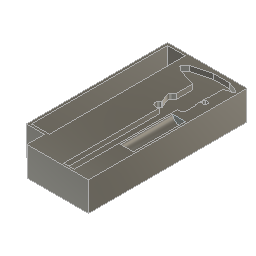
Dial-Caliper-Carrier (Autodesk Fusion 360 design; units mm, degrees)
Autodesk Fusion 360 part; units mm, degrees
(part 1 of 2)
sketch "Sketch1" plane through (0, 0, 3.175) normal (0, 0, 1) x (-1, 0, 0)
  line L0 (0, 0) -> (0, 297.942)
  line L1 (0, 297.942) -> (-407.924, 297.942)
  line L2 (-407.924, 297.942) -> (-407.924, 0)
  line L3 (-407.924, 0) -> (0, 0)
  line L4 (-407.924, 0) -> (-312.924, 0)
  line L5 (-312.924, 0) -> (-312.924, 245)
  line L6 (-312.924, 245) -> (-407.924, 245)
  line L7 (-407.924, 245) -> (-407.924, 0)
  dimension "d206" = 95
  dimension "d207" = 245
  constraint horizontal L4
  constraint vertical L5
  constraint horizontal L6
  constraint vertical L7
  constraint coincident L2.end L3.start
  measures "d206" distance of L2.end L4.end
  measures "d207" distance of L2.end L6.end
extrude "Extrude1" add sketch "Sketch1" along normal blind 45 contours L2 L3 L4 L5 L6 L7
sketch "Sketch2" plane through (0, 0, 48.175) normal (0, 0, 1) x (-1, 0, 0)
  line L0 (-407.924, 245) -> (-407.924, 0)
  line L1 (-407.924, 0) -> (-312.924, 0)
  line L2 (-312.924, 0) -> (-312.924, 245)
  line L3 (-312.924, 245) -> (-407.924, 245)
sketch "Sketch3" plane through (0, 0, 48.175) normal (0, 0, 1) x (-1, 0, 0)
  line L0 (-385.7159, 241.3097) -> (-385.7159, 82.3904)
  line L1 (-312.924, 245) -> (-407.924, 245)
  line L2 (-407.924, 245) -> (-407.924, 0)
  line L3 (-317.924, 240) -> (-317.924, 87.6)
  line L4 (-312.924, 0) -> (-312.924, 245)
  line L5 (-317.924, 87.6) -> (-336.974, 87.6)
  line L6 (-336.974, 87.6) -> (-336.974, 240)
  line L7 (-336.974, 240) -> (-317.924, 240)
  line L8 (-337.024, 240.05) -> (-317.874, 240.05)
  line L9 (-317.874, 240.05) -> (-317.874, 87.55)
  line L10 (-317.874, 87.55) -> (-337.024, 87.55)
  line L11 (-337.024, 87.55) -> (-337.024, 240.05)
  dimension "d210" = 152.4
  dimension "d211" = 5
  dimension "d212" = 5
  dimension "d213" = 19.05
  dimension "d214" = -0.05
  constraint parallel L0 L2
  constraint perpendicular L1 L3
  constraint perpendicular L3 L5
  constraint perpendicular L5 L6
  constraint perpendicular L3 L7
  measures "d210" distance of L3.start L3.end
  measures "d211" distance of L3 L4
  measures "d212" distance of L1 L3.start
  measures "d213" distance of L3.end L5.end
sketch "Sketch5" plane through (0, 0, 48.175) normal (0, 0, 1) x (-1, 0, 0)
  line L0 (-407.924, 245) -> (-407.924, 0)
  line L1 (-407.924, 0) -> (-312.924, 0)
  line L2 (-312.924, 0) -> (-312.924, 245)
  line L3 (-312.924, 245) -> (-407.924, 245)
  line L4 (-366.4147, 241.7185) -> (-366.3062, 93.0229)
  line L5 (-366.4147, 241.7185) -> (-382.673, 241.7066)
  line L6 (-382.673, 241.7066) -> (-382.5568, 82.4778)
  spline S0 degree 5 poles (-382.5568, 82.4778) (-382.5593, 82.4568) (-382.563, 82.4147) (-382.5646, 82.3519) (-382.559, 82.2687) (-382.5488, 82.169) (-382.5684, 82.0854) (-382.6594, 82.0319) (-382.8401, 82.0111) (-383.1037, 82.0144) (-383.4312, 82.0288) (-383.8005, 82.0428) (-384.1971, 82.0514) (-384.6109, 82.0543) (-385.0359, 82.0538) (-385.4676, 82.0533) (-385.9022, 82.0552) (-386.3345, 82.0591) (-386.7578, 82.0608) (-387.165, 82.0543) (-387.5495, 82.0319) (-387.9064, 81.9855) (-388.2336, 81.9077) (-388.5328, 81.7926) (-388.8079, 81.6362) (-389.0641, 81.4368) (-389.306, 81.1959) (-389.5364, 80.9182) (-389.7556, 80.6117) (-389.9622, 80.2849) (-390.1543, 79.9453) (-390.3301, 79.5967) (-390.4889, 79.2371) (-390.6319, 78.8575) (-390.7613, 78.4459) (-390.8799, 77.9908) (-390.9902, 77.4855) (-391.0939, 76.9317) (-391.1914, 76.3431) (-391.2811, 75.7505) (-391.3598, 75.1937) (-391.4238, 74.7122) (-391.4698, 74.337) (-391.4957, 74.0802) (-391.5015, 73.9279) (-391.4903, 73.827) (-391.4674, 73.701) (-391.4381, 73.482) (-391.4063, 73.1351) (-391.3744, 72.6507) (-391.344, 72.0401) (-391.3158, 71.3289) (-391.2898, 70.5518) (-391.2656, 69.7464) (-391.243, 68.9483) (-391.2214, 68.1843) (-391.2007, 67.4704) (-391.1809, 66.8139) (-391.1621, 66.2157) (-391.1444, 65.6712) (-391.1281, 65.1725) (-391.1133, 64.7103) (-391.1002, 64.2749) (-391.0891, 63.8589) (-391.0801, 63.4574) (-391.0732, 63.0673) (-391.0693, 62.7632) (-391.0674, 62.5394) (-391.0665, 62.3921) (-391.0662, 62.3189) knots 0 0 0 0 0 0 0.01538462 0.03076923 0.04615385 0.06153846 0.07692308 0.09230769 0.10769231 0.12307692 0.13846154 0.15384615 0.16923077 0.18461538 0.2 0.21538462 0.23076923 0.24615385 0.26153846 0.27692308 0.29230769 0.30769231 0.32307692 0.33846154 0.35384615 0.36923077 0.38461538 0.4 0.41538462 0.43076923 0.44615385 0.46153846 0.47692308 0.49230769 0.50769231 0.52307692 0.53846154 0.55384615 0.56923077 0.58461538 0.6 0.61538462 0.63076923 0.64615385 0.66153846 0.67692308 0.69230769 0.70769231 0.72307692 0.73846154 0.75384615 0.76923077 0.78461538 0.8 0.81538462 0.83076923 0.84615385 0.86153846 0.87692308 0.89230769 0.90769231 0.92307692 0.93846154 0.95384615 0.96923077 0.98461538 1 1 1 1 1 1
  spline S1 degree 5 poles (-389.9505, 61.1725) (-389.9505, 61.0932) (-389.9505, 60.9369) (-389.9505, 60.7095) (-389.9505, 60.42) (-389.9505, 60.0804) (-389.9505, 59.7592) (-389.9505, 59.4492) (-389.9505, 59.1366) (-389.9505, 58.8031) (-389.9505, 58.4302) (-389.9505, 58.0029) (-389.9505, 57.5144) (-389.9505, 56.97) (-389.9505, 56.385) (-389.9505, 55.7806) (-389.9505, 55.1811) (-389.9505, 54.6105) (-389.9505, 54.0894) (-389.9505, 53.6317) (-389.9505, 53.2443) (-389.9505, 52.993) (-389.9505, 52.8376) (-389.9505, 52.7487) (-389.9505, 52.7079) knots 0 0 0 0 0 0 0.05 0.1 0.15 0.2 0.25 0.3 0.35 0.4 0.45 0.5 0.55 0.6 0.65 0.7 0.75 0.8 0.85 0.9 0.95 1 1 1 1 1 1
  spline S2 degree 5 poles (-391.075, 63.1525) (-391.0747, 63.1374) (-391.0729, 63.1049) (-391.0668, 63.0492) (-391.0519, 62.9611) (-391.0219, 62.828) (-390.9803, 62.6732) (-390.927, 62.4996) (-390.8622, 62.3125) (-390.7861, 62.1204) (-390.6996, 61.933) (-390.6038, 61.7602) (-390.5004, 61.6101) (-390.3919, 61.4876) (-390.2816, 61.3926) (-390.1737, 61.3196) (-390.0836, 61.2661) (-390.0205, 61.2265) (-389.9798, 61.1969) (-389.9574, 61.1784) (-389.9505, 61.1725) knots 0 0 0 0 0 0 0.05 0.1 0.15 0.2 0.25 0.3 0.35 0.4 0.45 0.5 0.55 0.6 0.65 0.7 0.75 0.77292 0.77292 0.77292 0.77292 0.77292 0.77292
  line L7 (-390.106, 61.306) -> (-389.795, 61.0389)
  spline S3 degree 5 poles (-387.4662, 6.0325) (-386.4601, 6.0325) (-384.4479, 6.0325) (-381.4296, 6.0325) (-377.4051, 6.0325) (-372.3746, 6.0325) (-368.3502, 6.0325) (-365.3319, 6.0325) (-363.3197, 6.0325) (-362.3136, 6.0325) knots 0 0 0 0 0 0 0.2 0.4 0.6 0.8 1 1 1 1 1 1
  spline S4 degree 5 poles (-362.3136, 6.0325) (-362.1526, 6.0601) (-361.8173, 6.1205) (-361.274, 6.2265) (-360.4685, 6.3988) (-359.3264, 6.6655) (-358.0528, 6.9821) (-356.6573, 7.3442) (-355.1586, 7.7439) (-353.5804, 8.1713) (-351.9486, 8.6156) (-350.2888, 9.0666) (-348.6228, 9.5161) (-346.9663, 9.9592) (-345.3286, 10.394) (-343.7147, 10.8206) (-342.1264, 11.2407) (-340.5633, 11.6563) (-339.0245, 12.0695) (-337.5089, 12.4816) (-336.0158, 12.8932) (-334.8388, 13.2226) (-333.9657, 13.4696) (-333.3878, 13.6343) (-333.1, 13.7167) knots 0 0 0 0 0 0 0.05 0.1 0.15 0.2 0.25 0.3 0.35 0.4 0.45 0.5 0.55 0.6 0.65 0.7 0.75 0.8 0.85 0.9 0.95 1 1 1 1 1 1
  spline S5 degree 5 poles (-333.1, 13.7167) (-332.8186, 14.0144) (-332.2556, 14.6098) (-331.4112, 15.503) (-330.2854, 16.6939) (-328.8781, 18.1825) (-327.7522, 19.3734) (-326.9078, 20.2666) (-326.3449, 20.862) (-326.0635, 21.1597) knots 0 0 0 0 0 0 0.2 0.4 0.6 0.8 1 1 1 1 1 1
  spline S6 degree 5 poles (-326.0635, 21.1597) (-326.0507, 21.1722) (-326.0252, 21.197) (-325.9869, 21.2343) (-325.9359, 21.284) (-325.8721, 21.3461) (-325.821, 21.3957) (-325.7827, 21.433) (-325.7572, 21.4578) (-325.7445, 21.4703) knots 0 0 0 0 0 0 0.2 0.4 0.6 0.8 1 1 1 1 1 1
  spline S7 degree 5 poles (-332.3207, 27.7023) (-332.0446, 27.4406) (-331.4923, 26.9172) (-330.6638, 26.1321) (-329.5592, 25.0853) (-328.2439, 23.8389) (-327.2048, 22.8542) (-326.4419, 22.1312) (-325.9551, 21.6699) (-325.7445, 21.4703) knots 0 0 0 0 0 0 0.2 0.4 0.6 0.8 0.95254 0.95254 0.95254 0.95254 0.95254 0.95254
  line L8 (-326.4152, 22.1059) -> (-325.0737, 20.8346)
  line L9 (-332.3207, 27.7023) -> (-359.9697, 35.6695)
  line L10 (-359.9697, 35.6695) -> (-359.9697, 43.0263)
  line L11 (-359.9697, 43.0263) -> (-359.9697, 61.0097)
  spline S8 degree 5 poles (-359.9697, 61.0097) (-359.9018, 61.0819) (-359.7646, 61.2258) (-359.5543, 61.4403) (-359.2647, 61.7233) (-358.8875, 62.0728) (-358.4957, 62.4196) (-358.0905, 62.7671) (-357.674, 63.1207) (-357.2495, 63.4874) (-356.8218, 63.8741) (-356.3978, 64.2876) (-355.9865, 64.7329) (-355.5989, 65.2134) (-355.2464, 65.7307) (-354.9403, 66.2847) (-354.6905, 66.8732) (-354.5054, 67.4925) (-354.391, 68.1384) (-354.3516, 68.808) (-354.3894, 69.5005) (-354.5046, 70.219) (-354.6951, 70.9706) (-354.9569, 71.7634) (-355.2837, 72.6045) (-355.6671, 73.4983) (-356.0968, 74.4439) (-356.5602, 75.4327) (-357.0428, 76.4482) (-357.5291, 77.4686) (-358.0035, 78.4687) (-358.4508, 79.4224) (-358.8574, 80.3045) (-359.2118, 81.0929) (-359.5055, 81.771) (-359.7337, 82.3297) (-359.8622, 82.6775) (-359.9278, 82.8821) (-359.958, 82.9935) (-359.9697, 83.043) knots 0 0 0 0 0 0 0.028571 0.057143 0.085714 0.114286 0.142857 0.171429 0.2 0.228571 0.257143 0.285714 0.314286 0.342857 0.371429 0.4 0.428571 0.457143 0.485714 0.514286 0.542857 0.571429 0.6 0.628571 0.657143 0.685714 0.714286 0.742857 0.771429 0.8 0.828571 0.857143 0.885714 0.914286 0.942857 0.971429 1 1 1 1 1 1
  spline S9 degree 5 poles (-359.9697, 83.043) (-359.8778, 83.0783) (-359.6942, 83.1489) (-359.4187, 83.2549) (-359.0514, 83.3961) (-358.5923, 83.5727) (-358.2249, 83.7139) (-357.9495, 83.8198) (-357.7658, 83.8905) (-357.674, 83.9258) knots 0 0 0 0 0 0 0.2 0.4 0.6 0.8 1 1 1 1 1 1
  spline S10 degree 5 poles (-359.9697, 83.043) (-359.9166, 83.0639) (-359.81, 83.1056) (-359.6489, 83.1679) (-359.4317, 83.2503) (-359.1558, 83.3538) (-358.8752, 83.4625) (-358.5893, 83.5858) (-358.2969, 83.7381) (-357.9979, 83.9346) (-357.6939, 84.1868) (-357.389, 84.4988) (-357.091, 84.8639) (-356.8092, 85.2687) (-356.553, 85.6961) (-356.3303, 86.1297) (-356.1458, 86.5564) (-355.9991, 86.9709) (-355.8859, 87.3747) (-355.8004, 87.7738) (-355.7373, 88.1762) (-355.6936, 88.5902) (-355.6713, 89.0222) (-355.6759, 89.4755) (-355.7154, 89.9513) (-355.798, 90.4477) (-355.9313, 90.9599) (-356.1199, 91.4799) (-356.3653, 91.9969) (-356.6667, 92.4989) (-357.0208, 92.9738) (-357.4229, 93.4106) (-357.8674, 93.8004) (-358.3475, 94.1384) (-358.8567, 94.4239) (-359.3882, 94.6593) (-359.9353, 94.848) (-360.4919, 94.9934) (-361.0522, 95.0971) (-361.6114, 95.1576) (-362.1658, 95.1683) (-362.712, 95.1199) (-363.2471, 95.0039) (-363.7673, 94.8157) (-364.2682, 94.5576) (-364.7435, 94.2418) (-365.1849, 93.8948) (-365.5824, 93.5536) (-365.8932, 93.2873) (-366.0959, 93.134) (-366.2188, 93.0608) (-366.2846, 93.0312) (-366.3062, 93.0229) knots 0 0 0 0 0 0 0.02 0.04 0.06 0.08 0.1 0.12 0.14 0.16 0.18 0.2 0.22 0.24 0.26 0.28 0.3 0.32 0.34 0.36 0.38 0.4 0.42 0.44 0.46 0.48 0.5 0.52 0.54 0.56 0.58 0.6 0.62 0.64 0.66 0.68 0.7 0.72 0.74 0.76 0.78 0.8 0.82 0.84 0.86 0.88 0.9 0.92 0.94 0.950494 0.950494 0.950494 0.950494 0.950494 0.950494
  line L12 (-365.399, 93.3737) -> (-367.2134, 92.6721)
  line L13 (-387.8522, 7.1354) -> (-387.8522, 6.0325)
  line L14 (-387.8522, 6.0325) -> (-387.4662, 6.0325)
  line L15 (-387.8522, 6.8243) -> (-400.7794, 11.0064)
  line L16 (-400.7794, 11.0064) -> (-404.4624, 13.6097)
  line L17 (-404.4624, 13.6097) -> (-401.1196, 16.5087)
  line L18 (-401.1196, 16.5087) -> (-390.396, 19.9107)
  arc A0 (-390.396, 19.9107) -> (-390.6158, 20.6037) centre (-390.5059, 20.2572) ccw
  line L19 (-390.6158, 20.6037) -> (-390.6158, 41.3132)
  line L20 (-390.6158, 48.1829) -> (-396.3987, 48.1829)
  spline S11 degree 5 poles (-391.5467, 48.1829) (-391.5195, 48.185) (-391.4654, 48.1911) (-391.3847, 48.2058) (-391.2783, 48.2369) (-391.1473, 48.2953) (-391.0189, 48.374) (-390.8943, 48.4742) (-390.7753, 48.5968) (-390.6642, 48.7426) (-390.5636, 48.9124) (-390.4762, 49.1069) (-390.4037, 49.326) (-390.3474, 49.5695) (-390.3073, 49.8363) (-390.2832, 50.1256) (-390.2765, 50.3743) (-390.2784, 50.5702) (-390.2828, 50.705) (-390.2857, 50.7734) knots 0 0 0 0 0 0 0.066667 0.133333 0.2 0.266667 0.333333 0.4 0.466667 0.533333 0.6 0.666667 0.733333 0.8 0.866667 0.933333 1 1 1 1 1 1
  spline S12 degree 5 poles (-390.2857, 52.3633) (-390.2961, 52.4211) (-390.3173, 52.5354) (-390.3502, 52.7038) (-390.3967, 52.9217) (-390.4591, 53.1824) (-390.5263, 53.4305) (-390.5987, 53.6646) (-390.6766, 53.8841) (-390.7599, 54.0891) (-390.8482, 54.2808) (-390.9226, 54.4242) (-390.9803, 54.5265) (-391.0196, 54.5925) (-391.0395, 54.6249) knots 0 0 0 0 0 0 0.1 0.2 0.3 0.4 0.5 0.6 0.7 0.8 0.9 1 1 1 1 1 1
  spline S13 degree 5 poles (-391.0395, 54.6249) (-391.1432, 54.6249) (-391.3521, 54.6249) (-391.6698, 54.6249) (-392.102, 54.6249) (-392.6578, 54.6249) (-393.2304, 54.6249) (-393.8211, 54.6249) (-394.4301, 54.6249) (-395.0566, 54.6249) (-395.6991, 54.6249) (-396.2247, 54.6249) (-396.6251, 54.6249) (-396.8947, 54.6249) (-397.0302, 54.6249) knots 0 0 0 0 0 0 0.1 0.2 0.3 0.4 0.5 0.6 0.7 0.8 0.9 1 1 1 1 1 1
  spline S14 degree 5 poles (-397.0302, 54.6249) (-397.06, 54.605) (-397.1182, 54.5641) (-397.2016, 54.4991) (-397.3046, 54.4051) (-397.4199, 54.2753) (-397.5222, 54.1324) (-397.6123, 53.9753) (-397.6921, 53.8022) (-397.7634, 53.611) (-397.8286, 53.3999) (-397.8892, 53.168) (-397.946, 52.916) (-397.9988, 52.6463) (-398.0463, 52.3623) (-398.0869, 52.0681) (-398.1183, 51.7675) (-398.1381, 51.4639) (-398.1438, 51.1591) (-398.1331, 50.8546) (-398.104, 50.551) (-398.0548, 50.2496) (-397.9848, 49.952) (-397.8939, 49.6613) (-397.7831, 49.3821) (-397.6541, 49.1201) (-397.5092, 48.8811) (-397.3504, 48.6711) (-397.1797, 48.4948) (-396.9988, 48.3556) (-396.8084, 48.2552) (-396.6489, 48.2065) (-396.5253, 48.1877) (-396.4412, 48.1832) (-396.3987, 48.1829) knots 0 0 0 0 0 0 0.033333 0.066667 0.1 0.133333 0.166667 0.2 0.233333 0.266667 0.3 0.333333 0.366667 0.4 0.433333 0.466667 0.5 0.533333 0.566667 0.6 0.633333 0.666667 0.7 0.733333 0.766667 0.8 0.833333 0.866667 0.9 0.933333 0.966667 1 1 1 1 1 1
  line L21 (-390.2857, 50.7734) -> (-389.869, 50.7734)
  line L22 (-389.869, 50.7734) -> (-389.869, 42.5841)
  line L23 (-389.869, 42.5841) -> (-390.6158, 41.3132)
  line L24 (-390.2857, 52.3633) -> (-389.9496, 52.3633)
  line L25 (-389.9496, 52.3633) -> (-389.9505, 52.7079)
  point P0 (-382.5566, 82.2421)
  point P1 (-382.6149, 82.068)
  point P2 (-383.4158, 82.0278)
  point P3 (-385.6935, 82.0546)
  point P4 (-387.9176, 81.9742)
  point P5 (-389.2173, 81.2775)
  point P6 (-390.3025, 79.6429)
  point P7 (-391.1064, 76.8426)
  point P8 (-391.495, 74.0424)
  point P9 (-391.4682, 73.6941)
  point P10 (-391.2538, 69.3262)
  point P11 (-391.1064, 64.4761)
  point P12 (-390.9289, 62.5109)
  point P13 (-390.428, 61.5325)
  point P14 (-389.9505, 59.6047)
  point P15 (-389.9505, 57.9413)
  point P16 (-389.9505, 54.4545)
  point P17 (-358.1946, 6.9498)
  point P18 (-349.922, 9.165)
  point P19 (-340.888, 11.5706)
  point P20 (-358.509, 62.4052)
  point P21 (-356.7435, 63.956)
  point P22 (-355.0257, 66.151)
  point P23 (-354.3815, 69.1811)
  point P24 (-355.9084, 74.0244)
  point P25 (-359.1532, 80.9673)
  point P26 (-358.9561, 83.4328)
  point P27 (-357.7318, 84.1668)
  point P28 (-356.2907, 86.2339)
  point P29 (-355.7325, 88.2562)
  point P30 (-355.8698, 90.6995)
  point P31 (-357.7915, 93.7193)
  point P32 (-361.159, 95.1011)
  point P33 (-364.3984, 94.4606)
  point P34 (-390.971, 48.4159)
  point P35 (-390.4638, 49.156)
  point P36 (-390.6154, 53.7066)
  point P37 (-393.7051, 54.6249)
  point P38 (-397.5325, 54.1077)
  point P39 (-397.8674, 53.2466)
  point P40 (-398.1186, 51.7276)
  point P41 (-397.987, 49.9813)
  point P42 (-397.2813, 48.6058)
  constraint perpendicular L4 L5
  constraint perpendicular L5 L6
  constraint coincident S0 S2.start
  constraint coincident S1.start S2.end
  constraint midpoint S1.start L7
  constraint midpoint S6.end L8
  constraint vertical L10
  constraint parallel L10 L11
  constraint coincident S9 P26
  constraint midpoint L4.end L12
  constraint vertical L13
  constraint perpendicular L13 L14
  constraint coincident L13 L15.start
  constraint tangent L18 A0
  constraint vertical L19
  constraint perpendicular L19 L20
  constraint coincident L20 S11.start
  constraint horizontal L21
  constraint perpendicular L21 L22
  constraint perpendicular L19 L24
extrude "Extrude4" cut sketch "Sketch5" against normal blind 8 contours L4 L5 L6 S0 S1 S2 S3 S4 S5 S6 S7 L8 L9 L10 L11 S8 S10 L13 L14 L15 L16 L17 L18 A0 L19 L20 S11 S12 S13 S14 L21 L22 L23 L24 L25
sketch "Sketch11" plane through (0, 0, 48.175) normal (0, 0, 1) x (-1, 0, 0)
  line L0 (-362.3136, 6.0325) -> (-387.8522, 6.0325)
  line L1 (-387.8522, 6.0325) -> (-387.8522, 6.8243)
  line L2 (-387.8522, 6.8243) -> (-400.7794, 11.0064)
  line L3 (-400.7794, 11.0064) -> (-404.4624, 13.6097)
  line L4 (-404.4624, 13.6097) -> (-401.1196, 16.5087)
  line L5 (-401.1196, 16.5087) -> (-390.396, 19.9107)
  arc A0 (-390.396, 19.9107) -> (-390.6158, 20.6037) centre (-390.5059, 20.2572) ccw
  line L6 (-390.6158, 20.6037) -> (-390.6158, 41.3132)
  line L7 (-390.6158, 41.3132) -> (-389.869, 42.5841)
  line L8 (-389.869, 42.5841) -> (-389.869, 50.7734)
  line L9 (-389.869, 50.7734) -> (-390.2857, 50.7734)
  spline S0 degree 5 poles (-390.2857, 50.7734) (-390.2828, 50.705) (-390.2784, 50.5702) (-390.2765, 50.3743) (-390.2832, 50.1256) (-390.3073, 49.8363) (-390.3474, 49.5695) (-390.4037, 49.326) (-390.4762, 49.1069) (-390.5636, 48.9124) (-390.6642, 48.7426) (-390.7753, 48.5968) (-390.8943, 48.4742) (-391.0189, 48.374) (-391.1473, 48.2953) (-391.2783, 48.2369) (-391.3847, 48.2058) (-391.4654, 48.1911) (-391.5195, 48.185) (-391.5467, 48.1829) knots -1 -1 -1 -1 -1 -1 -0.933333 -0.866667 -0.8 -0.733333 -0.666667 -0.6 -0.533333 -0.466667 -0.4 -0.333333 -0.266667 -0.2 -0.133333 -0.066667 0 0 0 0 0 0
  line L10 (-391.5467, 48.1829) -> (-396.3987, 48.1829)
  spline S1 degree 5 poles (-396.3987, 48.1829) (-396.4412, 48.1832) (-396.5253, 48.1877) (-396.6489, 48.2065) (-396.8084, 48.2552) (-396.9988, 48.3556) (-397.1797, 48.4948) (-397.3504, 48.6711) (-397.5092, 48.8811) (-397.6541, 49.1201) (-397.7831, 49.3821) (-397.8939, 49.6613) (-397.9848, 49.952) (-398.0548, 50.2496) (-398.104, 50.551) (-398.1331, 50.8546) (-398.1438, 51.1591) (-398.1381, 51.4639) (-398.1183, 51.7675) (-398.0869, 52.0681) (-398.0463, 52.3623) (-397.9988, 52.6463) (-397.946, 52.916) (-397.8892, 53.168) (-397.8286, 53.3999) (-397.7634, 53.611) (-397.6921, 53.8022) (-397.6123, 53.9753) (-397.5222, 54.1324) (-397.4199, 54.2753) (-397.3046, 54.4051) (-397.2016, 54.4991) (-397.1182, 54.5641) (-397.06, 54.605) (-397.0302, 54.6249) knots -1 -1 -1 -1 -1 -1 -0.966667 -0.933333 -0.9 -0.866667 -0.833333 -0.8 -0.766667 -0.733333 -0.7 -0.666667 -0.633333 -0.6 -0.566667 -0.533333 -0.5 -0.466667 -0.433333 -0.4 -0.366667 -0.333333 -0.3 -0.266667 -0.233333 -0.2 -0.166667 -0.133333 -0.1 -0.066667 -0.033333 0 0 0 0 0 0
  line L11 (-397.0302, 54.6249) -> (-391.0395, 54.6249)
  spline S2 degree 5 poles (-391.0395, 54.6249) (-391.0196, 54.5925) (-390.9803, 54.5265) (-390.9226, 54.4242) (-390.8482, 54.2808) (-390.7599, 54.0891) (-390.6766, 53.8841) (-390.5987, 53.6646) (-390.5263, 53.4305) (-390.4591, 53.1824) (-390.3967, 52.9217) (-390.3502, 52.7038) (-390.3173, 52.5354) (-390.2961, 52.4211) (-390.2857, 52.3633) knots -1 -1 -1 -1 -1 -1 -0.9 -0.8 -0.7 -0.6 -0.5 -0.4 -0.3 -0.2 -0.1 0 0 0 0 0 0
  line L12 (-390.2857, 52.3633) -> (-389.9496, 52.3633)
  line L13 (-389.9496, 52.3633) -> (-389.9505, 52.7079)
  line L14 (-389.9505, 52.7079) -> (-389.9505, 61.1725)
  spline S3 degree 5 poles (-389.9505, 61.1725) (-389.9574, 61.1784) (-389.9798, 61.1969) (-390.0205, 61.2265) (-390.0836, 61.2661) (-390.1737, 61.3196) (-390.2816, 61.3926) (-390.3919, 61.4876) (-390.5004, 61.6101) (-390.6038, 61.7602) (-390.6996, 61.933) (-390.7861, 62.1204) (-390.8622, 62.3125) (-390.927, 62.4996) (-390.9803, 62.6732) (-391.0219, 62.828) (-391.0519, 62.9611) (-391.0668, 63.0492) (-391.0729, 63.1049) (-391.0747, 63.1374) (-391.075, 63.1525) knots -0.77292 -0.77292 -0.77292 -0.77292 -0.77292 -0.77292 -0.75 -0.7 -0.65 -0.6 -0.55 -0.5 -0.45 -0.4 -0.35 -0.3 -0.25 -0.2 -0.15 -0.1 -0.05 0 0 0 0 0 0
  spline S4 degree 5 poles (-391.075, 63.1525) (-391.076, 63.2134) (-391.0784, 63.3525) (-391.0827, 63.5721) (-391.0896, 63.8767) (-391.1002, 64.2749) (-391.1133, 64.7103) (-391.1281, 65.1725) (-391.1444, 65.6712) (-391.1621, 66.2157) (-391.1809, 66.8139) (-391.2007, 67.4704) (-391.2214, 68.1843) (-391.243, 68.9483) (-391.2656, 69.7464) (-391.2898, 70.5518) (-391.3158, 71.3289) (-391.344, 72.0401) (-391.3744, 72.6507) (-391.4063, 73.1351) (-391.4381, 73.482) (-391.4674, 73.701) (-391.4903, 73.827) (-391.5015, 73.9279) (-391.4957, 74.0802) (-391.4698, 74.337) (-391.4238, 74.7122) (-391.3598, 75.1937) (-391.2811, 75.7505) (-391.1914, 76.3431) (-391.0939, 76.9317) (-390.9902, 77.4855) (-390.8799, 77.9908) (-390.7613, 78.4459) (-390.6319, 78.8575) (-390.4889, 79.2371) (-390.3301, 79.5967) (-390.1543, 79.9453) (-389.9622, 80.2849) (-389.7556, 80.6117) (-389.5364, 80.9182) (-389.306, 81.1959) (-389.0641, 81.4368) (-388.8079, 81.6362) (-388.5328, 81.7926) (-388.2336, 81.9077) (-387.9064, 81.9855) (-387.5495, 82.0319) (-387.165, 82.0543) (-386.7578, 82.0608) (-386.3345, 82.0591) (-385.9022, 82.0552) (-385.4676, 82.0533) (-385.0359, 82.0538) (-384.6109, 82.0543) (-384.1971, 82.0514) (-383.8005, 82.0428) (-383.4312, 82.0288) (-383.1037, 82.0144) (-382.8401, 82.0111) (-382.6594, 82.0319) (-382.5684, 82.0854) (-382.5488, 82.169) (-382.559, 82.2687) (-382.5646, 82.3519) (-382.563, 82.4147) (-382.5593, 82.4568) (-382.5568, 82.4778) knots -0.96593682 -0.96593682 -0.96593682 -0.96593682 -0.96593682 -0.96593682 -0.95384615 -0.93846154 -0.92307692 -0.90769231 -0.89230769 -0.87692308 -0.86153846 -0.84615385 -0.83076923 -0.81538462 -0.8 -0.78461538 -0.76923077 -0.75384615 -0.73846154 -0.72307692 -0.70769231 -0.69230769 -0.67692308 -0.66153846 -0.64615385 -0.63076923 -0.61538462 -0.6 -0.58461538 -0.56923077 -0.55384615 -0.53846154 -0.52307692 -0.50769231 -0.49230769 -0.47692308 -0.46153846 -0.44615385 -0.43076923 -0.41538462 -0.4 -0.38461538 -0.36923077 -0.35384615 -0.33846154 -0.32307692 -0.30769231 -0.29230769 -0.27692308 -0.26153846 -0.24615385 -0.23076923 -0.21538462 -0.2 -0.18461538 -0.16923077 -0.15384615 -0.13846154 -0.12307692 -0.10769231 -0.09230769 -0.07692308 -0.06153846 -0.04615385 -0.03076923 -0.01538462 0 0 0 0 0 0
  line L15 (-382.5568, 82.4778) -> (-382.673, 241.7066)
  line L16 (-382.673, 241.7066) -> (-366.4147, 241.7185)
  line L17 (-366.4147, 241.7185) -> (-366.3062, 93.0229)
  spline S5 degree 5 poles (-366.3062, 93.0229) (-366.2846, 93.0312) (-366.2188, 93.0608) (-366.0959, 93.134) (-365.8932, 93.2873) (-365.5824, 93.5536) (-365.1849, 93.8948) (-364.7435, 94.2418) (-364.2682, 94.5576) (-363.7673, 94.8157) (-363.2471, 95.0039) (-362.712, 95.1199) (-362.1658, 95.1683) (-361.6114, 95.1576) (-361.0522, 95.0971) (-360.4919, 94.9934) (-359.9353, 94.848) (-359.3882, 94.6593) (-358.8567, 94.4239) (-358.3475, 94.1384) (-357.8674, 93.8004) (-357.4229, 93.4106) (-357.0208, 92.9738) (-356.6667, 92.4989) (-356.3653, 91.9969) (-356.1199, 91.4799) (-355.9313, 90.9599) (-355.798, 90.4477) (-355.7154, 89.9513) (-355.6759, 89.4755) (-355.6713, 89.0222) (-355.6936, 88.5902) (-355.7373, 88.1762) (-355.8004, 87.7738) (-355.8859, 87.3747) (-355.9991, 86.9709) (-356.1458, 86.5564) (-356.3303, 86.1297) (-356.553, 85.6961) (-356.8092, 85.2687) (-357.091, 84.8639) (-357.389, 84.4988) (-357.6939, 84.1868) (-357.9979, 83.9346) (-358.2969, 83.7381) (-358.5478, 83.6074) (-358.7368, 83.5228) (-358.8668, 83.4687) (-358.9397, 83.4393) (-358.9561, 83.4328) knots -0.950494 -0.950494 -0.950494 -0.950494 -0.950494 -0.950494 -0.94 -0.92 -0.9 -0.88 -0.86 -0.84 -0.82 -0.8 -0.78 -0.76 -0.74 -0.72 -0.7 -0.68 -0.66 -0.64 -0.62 -0.6 -0.58 -0.56 -0.54 -0.52 -0.5 -0.48 -0.46 -0.44 -0.42 -0.4 -0.38 -0.36 -0.34 -0.32 -0.3 -0.28 -0.26 -0.24 -0.22 -0.2 -0.18 -0.16 -0.14 -0.12 -0.1 -0.08 -0.074178 -0.074178 -0.074178 -0.074178 -0.074178 -0.074178
  line L18 (-358.9561, 83.4328) -> (-359.4097, 83.2583)
  spline S6 degree 5 poles (-359.4097, 83.2583) (-359.4139, 83.2568) (-359.4729, 83.2345) (-359.5862, 83.1916) (-359.6985, 83.1487) (-359.81, 83.1056) (-359.9166, 83.0639) (-359.9697, 83.043) knots -0.041525 -0.041525 -0.041525 -0.041525 -0.041525 -0.041525 -0.04 -0.02 0 0 0 0 0 0
  spline S7 degree 5 poles (-359.9697, 83.043) (-359.958, 82.9935) (-359.9278, 82.8821) (-359.8622, 82.6775) (-359.7337, 82.3297) (-359.5055, 81.771) (-359.2118, 81.0929) (-358.8574, 80.3045) (-358.4508, 79.4224) (-358.0035, 78.4687) (-357.5291, 77.4686) (-357.0428, 76.4482) (-356.5602, 75.4327) (-356.0968, 74.4439) (-355.6671, 73.4983) (-355.2837, 72.6045) (-354.9569, 71.7634) (-354.6951, 70.9706) (-354.5046, 70.219) (-354.3894, 69.5005) (-354.3516, 68.808) (-354.391, 68.1384) (-354.5054, 67.4925) (-354.6905, 66.8732) (-354.9403, 66.2847) (-355.2464, 65.7307) (-355.5989, 65.2134) (-355.9865, 64.7329) (-356.3978, 64.2876) (-356.8218, 63.8741) (-357.2495, 63.4874) (-357.674, 63.1207) (-358.0905, 62.7671) (-358.4957, 62.4196) (-358.8875, 62.0728) (-359.2647, 61.7233) (-359.5543, 61.4403) (-359.7646, 61.2258) (-359.9018, 61.0819) (-359.9697, 61.0097) knots -1 -1 -1 -1 -1 -1 -0.971429 -0.942857 -0.914286 -0.885714 -0.857143 -0.828571 -0.8 -0.771429 -0.742857 -0.714286 -0.685714 -0.657143 -0.628571 -0.6 -0.571429 -0.542857 -0.514286 -0.485714 -0.457143 -0.428571 -0.4 -0.371429 -0.342857 -0.314286 -0.285714 -0.257143 -0.228571 -0.2 -0.171429 -0.142857 -0.114286 -0.085714 -0.057143 -0.028571 0 0 0 0 0 0
  line L19 (-359.9697, 61.0097) -> (-359.9697, 35.6695)
  line L20 (-359.9697, 35.6695) -> (-332.3207, 27.7023)
  line L21 (-332.3207, 27.7023) -> (-325.7445, 21.4703)
  line L22 (-325.7445, 21.4703) -> (-326.0635, 21.1597)
  line L23 (-326.0635, 21.1597) -> (-333.1, 13.7167)
  spline S8 degree 5 poles (-333.1, 13.7167) (-333.3878, 13.6343) (-333.9657, 13.4696) (-334.8388, 13.2226) (-336.0158, 12.8932) (-337.5089, 12.4816) (-339.0245, 12.0695) (-340.5633, 11.6563) (-342.1264, 11.2407) (-343.7147, 10.8206) (-345.3286, 10.394) (-346.9663, 9.9592) (-348.6228, 9.5161) (-350.2888, 9.0666) (-351.9486, 8.6156) (-353.5804, 8.1713) (-355.1586, 7.7439) (-356.6573, 7.3442) (-358.0528, 6.9821) (-359.3264, 6.6655) (-360.4685, 6.3988) (-361.274, 6.2265) (-361.8173, 6.1205) (-362.1526, 6.0601) (-362.3136, 6.0325) knots -1 -1 -1 -1 -1 -1 -0.95 -0.9 -0.85 -0.8 -0.75 -0.7 -0.65 -0.6 -0.55 -0.5 -0.45 -0.4 -0.35 -0.3 -0.25 -0.2 -0.15 -0.1 -0.05 0 0 0 0 0 0
  line L24 (-407.924, 245) -> (-407.924, 0)
  line L25 (-407.924, 0) -> (-312.924, 0)
  line L26 (-312.924, 0) -> (-312.924, 245)
  line L27 (-312.924, 245) -> (-407.924, 245)
  line L28 (-351.7415, 101.5229) -> (-371.5415, 101.5229)
  dimension "d224" = 19.8
  dimension "d227" = 8.5
  dimension "d229" = 5.2291
  dimension "d230" = 143.4771
  constraint horizontal L28
  measures "d224" distance of L28.start L28.end
  measures "d227" distance of L17.end L28
  measures "d229" distance of L17 L28.end
  measures "d230" distance of L27 L28
ref_plane "WorkPlane2" through (360.424, -92, 25.675) normal (0, -1, 0) x (1, 0, 0)
sketch "Sketch7" plane through (0, -92, 0) normal (0, -1, 0) x (-1, 0, 0)
  line L0 (-312.924, -48.175) -> (-407.924, -48.175)
  circle A0 centre (-395.0102, -48.175) radius 9.9
  dimension "d234" = 19.8
  constraint coincident L0 A0.centre
  measures "d234" diameter of A0
extrude "Extrude6" cut sketch "Sketch7" along normal blind 80.6
sketch "Sketch8" plane through (0, -92, 0) normal (0, -1, 0) x (1, 0, 0)
  line L0 (404.9102, 48.175) -> (385.1102, 48.175)
  arc A0 (385.1102, 48.175) -> (404.9102, 48.175) centre (395.0102, 48.175) ccw
sketch "Sketch9" plane through (0, 0, 3.175) normal (0, 0, 1) x (-1, 0, 0)
  line L0 (0, 0) -> (0, 297.942)
  line L1 (0, 297.942) -> (-407.924, 297.942)
  line L2 (-407.924, 297.942) -> (-407.924, 0)
  line L3 (-407.924, 0) -> (0, 0)
  line L4 (-312.924, 0) -> (-312.924, 245)
  line L5 (-285.1, 177.942) -> (-285.1, 0)
  line L6 (-312.924, 0) -> (-285.1, 0)
  line L7 (-285.1, 0) -> (-285.1, 220)
  line L8 (-285.1, 220) -> (-312.924, 220)
  line L9 (-312.924, 220) -> (-312.924, 0)
  dimension "d237" = 220
  constraint horizontal L6
  constraint vertical L7
  constraint horizontal L8
  constraint vertical L9
  constraint coincident L4.start L6.start
  measures "d237" distance of L4.start L8.end
extrude "Extrude7" add sketch "Sketch9" along normal blind 45 contours L3 L4 L5 L6 L7 L8 L9
sketch "Sketch10" plane through (0, 0, 48.175) normal (0, 0, 1) x (-1, 0, 0)
  line L0 (-404.9102, 92) -> (-404.9102, 172.6)
  line L1 (-404.9102, 172.6) -> (-385.1102, 172.6)
  line L2 (-385.1102, 172.6) -> (-385.1102, 92)
  line L3 (-385.1102, 92) -> (-404.9102, 92)
  line L4 (-362.3136, 6.0325) -> (-387.8522, 6.0325)
  line L5 (-387.8522, 6.0325) -> (-387.8522, 6.8243)
  line L6 (-387.8522, 6.8243) -> (-400.7794, 11.0064)
  line L7 (-400.7794, 11.0064) -> (-404.4624, 13.6097)
  line L8 (-404.4624, 13.6097) -> (-401.1196, 16.5087)
  line L9 (-401.1196, 16.5087) -> (-390.396, 19.9107)
  arc A0 (-390.396, 19.9107) -> (-390.6158, 20.6037) centre (-390.5059, 20.2572) ccw
  line L10 (-390.6158, 20.6037) -> (-390.6158, 41.3132)
  line L11 (-390.6158, 41.3132) -> (-389.869, 42.5841)
  line L12 (-389.869, 42.5841) -> (-389.869, 50.7734)
  line L13 (-389.869, 50.7734) -> (-390.2857, 50.7734)
  spline S0 degree 5 poles (-390.2857, 50.7734) (-390.2828, 50.705) (-390.2784, 50.5702) (-390.2765, 50.3743) (-390.2832, 50.1256) (-390.3073, 49.8363) (-390.3474, 49.5695) (-390.4037, 49.326) (-390.4762, 49.1069) (-390.5636, 48.9124) (-390.6642, 48.7426) (-390.7753, 48.5968) (-390.8943, 48.4742) (-391.0189, 48.374) (-391.1473, 48.2953) (-391.2783, 48.2369) (-391.3847, 48.2058) (-391.4654, 48.1911) (-391.5195, 48.185) (-391.5467, 48.1829) knots -1 -1 -1 -1 -1 -1 -0.933333 -0.866667 -0.8 -0.733333 -0.666667 -0.6 -0.533333 -0.466667 -0.4 -0.333333 -0.266667 -0.2 -0.133333 -0.066667 0 0 0 0 0 0
  line L14 (-391.5467, 48.1829) -> (-396.3987, 48.1829)
  spline S1 degree 5 poles (-396.3987, 48.1829) (-396.4412, 48.1832) (-396.5253, 48.1877) (-396.6489, 48.2065) (-396.8084, 48.2552) (-396.9988, 48.3556) (-397.1797, 48.4948) (-397.3504, 48.6711) (-397.5092, 48.8811) (-397.6541, 49.1201) (-397.7831, 49.3821) (-397.8939, 49.6613) (-397.9848, 49.952) (-398.0548, 50.2496) (-398.104, 50.551) (-398.1331, 50.8546) (-398.1438, 51.1591) (-398.1381, 51.4639) (-398.1183, 51.7675) (-398.0869, 52.0681) (-398.0463, 52.3623) (-397.9988, 52.6463) (-397.946, 52.916) (-397.8892, 53.168) (-397.8286, 53.3999) (-397.7634, 53.611) (-397.6921, 53.8022) (-397.6123, 53.9753) (-397.5222, 54.1324) (-397.4199, 54.2753) (-397.3046, 54.4051) (-397.2016, 54.4991) (-397.1182, 54.5641) (-397.06, 54.605) (-397.0302, 54.6249) knots -1 -1 -1 -1 -1 -1 -0.966667 -0.933333 -0.9 -0.866667 -0.833333 -0.8 -0.766667 -0.733333 -0.7 -0.666667 -0.633333 -0.6 -0.566667 -0.533333 -0.5 -0.466667 -0.433333 -0.4 -0.366667 -0.333333 -0.3 -0.266667 -0.233333 -0.2 -0.166667 -0.133333 -0.1 -0.066667 -0.033333 0 0 0 0 0 0
  line L15 (-397.0302, 54.6249) -> (-391.0395, 54.6249)
  spline S2 degree 5 poles (-391.0395, 54.6249) (-391.0196, 54.5925) (-390.9803, 54.5265) (-390.9226, 54.4242) (-390.8482, 54.2808) (-390.7599, 54.0891) (-390.6766, 53.8841) (-390.5987, 53.6646) (-390.5263, 53.4305) (-390.4591, 53.1824) (-390.3967, 52.9217) (-390.3502, 52.7038) (-390.3173, 52.5354) (-390.2961, 52.4211) (-390.2857, 52.3633) knots -1 -1 -1 -1 -1 -1 -0.9 -0.8 -0.7 -0.6 -0.5 -0.4 -0.3 -0.2 -0.1 0 0 0 0 0 0
  line L16 (-390.2857, 52.3633) -> (-389.9496, 52.3633)
  line L17 (-389.9496, 52.3633) -> (-389.9505, 52.7079)
  line L18 (-389.9505, 52.7079) -> (-389.9505, 61.1725)
  spline S3 degree 5 poles (-389.9505, 61.1725) (-389.9574, 61.1784) (-389.9798, 61.1969) (-390.0205, 61.2265) (-390.0836, 61.2661) (-390.1737, 61.3196) (-390.2816, 61.3926) (-390.3919, 61.4876) (-390.5004, 61.6101) (-390.6038, 61.7602) (-390.6996, 61.933) (-390.7861, 62.1204) (-390.8622, 62.3125) (-390.927, 62.4996) (-390.9803, 62.6732) (-391.0219, 62.828) (-391.0519, 62.9611) (-391.0668, 63.0492) (-391.0729, 63.1049) (-391.0747, 63.1374) (-391.075, 63.1525) knots -0.77292 -0.77292 -0.77292 -0.77292 -0.77292 -0.77292 -0.75 -0.7 -0.65 -0.6 -0.55 -0.5 -0.45 -0.4 -0.35 -0.3 -0.25 -0.2 -0.15 -0.1 -0.05 0 0 0 0 0 0
  spline S4 degree 5 poles (-391.075, 63.1525) (-391.076, 63.2134) (-391.0784, 63.3525) (-391.0827, 63.5721) (-391.0896, 63.8767) (-391.1002, 64.2749) (-391.1133, 64.7103) (-391.1281, 65.1725) (-391.1444, 65.6712) (-391.1621, 66.2157) (-391.1809, 66.8139) (-391.2007, 67.4704) (-391.2214, 68.1843) (-391.243, 68.9483) (-391.2656, 69.7464) (-391.2898, 70.5518) (-391.3158, 71.3289) (-391.344, 72.0401) (-391.3744, 72.6507) (-391.4063, 73.1351) (-391.4381, 73.482) (-391.4674, 73.701) (-391.4903, 73.827) (-391.5015, 73.9279) (-391.4957, 74.0802) (-391.4698, 74.337) (-391.4238, 74.7122) (-391.3598, 75.1937) (-391.2811, 75.7505) (-391.1914, 76.3431) (-391.0939, 76.9317) (-390.9902, 77.4855) (-390.8799, 77.9908) (-390.7613, 78.4459) (-390.6319, 78.8575) (-390.4889, 79.2371) (-390.3301, 79.5967) (-390.1543, 79.9453) (-389.9622, 80.2849) (-389.7556, 80.6117) (-389.5364, 80.9182) (-389.306, 81.1959) (-389.0641, 81.4368) (-388.8079, 81.6362) (-388.5328, 81.7926) (-388.2336, 81.9077) (-387.9064, 81.9855) (-387.5495, 82.0319) (-387.165, 82.0543) (-386.7578, 82.0608) (-386.3345, 82.0591) (-385.9022, 82.0552) (-385.4676, 82.0533) (-385.0359, 82.0538) (-384.6109, 82.0543) (-384.1971, 82.0514) (-383.8005, 82.0428) (-383.4312, 82.0288) (-383.1037, 82.0144) (-382.8401, 82.0111) (-382.6594, 82.0319) (-382.5684, 82.0854) (-382.5488, 82.169) (-382.559, 82.2687) (-382.5646, 82.3519) (-382.563, 82.4147) (-382.5593, 82.4568) (-382.5568, 82.4778) knots -0.96593682 -0.96593682 -0.96593682 -0.96593682 -0.96593682 -0.96593682 -0.95384615 -0.93846154 -0.92307692 -0.90769231 -0.89230769 -0.87692308 -0.86153846 -0.84615385 -0.83076923 -0.81538462 -0.8 -0.78461538 -0.76923077 -0.75384615 -0.73846154 -0.72307692 -0.70769231 -0.69230769 -0.67692308 -0.66153846 -0.64615385 -0.63076923 -0.61538462 -0.6 -0.58461538 -0.56923077 -0.55384615 -0.53846154 -0.52307692 -0.50769231 -0.49230769 -0.47692308 -0.46153846 -0.44615385 -0.43076923 -0.41538462 -0.4 -0.38461538 -0.36923077 -0.35384615 -0.33846154 -0.32307692 -0.30769231 -0.29230769 -0.27692308 -0.26153846 -0.24615385 -0.23076923 -0.21538462 -0.2 -0.18461538 -0.16923077 -0.15384615 -0.13846154 -0.12307692 -0.10769231 -0.09230769 -0.07692308 -0.06153846 -0.04615385 -0.03076923 -0.01538462 0 0 0 0 0 0
  line L19 (-382.5568, 82.4778) -> (-382.673, 241.7066)
  line L20 (-382.673, 241.7066) -> (-366.4147, 241.7185)
  line L21 (-366.4147, 241.7185) -> (-366.3062, 93.0229)
  spline S5 degree 5 poles (-366.3062, 93.0229) (-366.2846, 93.0312) (-366.2188, 93.0608) (-366.0959, 93.134) (-365.8932, 93.2873) (-365.5824, 93.5536) (-365.1849, 93.8948) (-364.7435, 94.2418) (-364.2682, 94.5576) (-363.7673, 94.8157) (-363.2471, 95.0039) (-362.712, 95.1199) (-362.1658, 95.1683) (-361.6114, 95.1576) (-361.0522, 95.0971) (-360.4919, 94.9934) (-359.9353, 94.848) (-359.3882, 94.6593) (-358.8567, 94.4239) (-358.3475, 94.1384) (-357.8674, 93.8004) (-357.4229, 93.4106) (-357.0208, 92.9738) (-356.6667, 92.4989) (-356.3653, 91.9969) (-356.1199, 91.4799) (-355.9313, 90.9599) (-355.798, 90.4477) (-355.7154, 89.9513) (-355.6759, 89.4755) (-355.6713, 89.0222) (-355.6936, 88.5902) (-355.7373, 88.1762) (-355.8004, 87.7738) (-355.8859, 87.3747) (-355.9991, 86.9709) (-356.1458, 86.5564) (-356.3303, 86.1297) (-356.553, 85.6961) (-356.8092, 85.2687) (-357.091, 84.8639) (-357.389, 84.4988) (-357.6939, 84.1868) (-357.9979, 83.9346) (-358.2969, 83.7381) (-358.5478, 83.6074) (-358.7368, 83.5228) (-358.8668, 83.4687) (-358.9397, 83.4393) (-358.9561, 83.4328) knots -0.950494 -0.950494 -0.950494 -0.950494 -0.950494 -0.950494 -0.94 -0.92 -0.9 -0.88 -0.86 -0.84 -0.82 -0.8 -0.78 -0.76 -0.74 -0.72 -0.7 -0.68 -0.66 -0.64 -0.62 -0.6 -0.58 -0.56 -0.54 -0.52 -0.5 -0.48 -0.46 -0.44 -0.42 -0.4 -0.38 -0.36 -0.34 -0.32 -0.3 -0.28 -0.26 -0.24 -0.22 -0.2 -0.18 -0.16 -0.14 -0.12 -0.1 -0.08 -0.074178 -0.074178 -0.074178 -0.074178 -0.074178 -0.074178
  line L22 (-358.9561, 83.4328) -> (-359.4097, 83.2583)
  spline S6 degree 5 poles (-359.4097, 83.2583) (-359.4139, 83.2568) (-359.4729, 83.2345) (-359.5862, 83.1916) (-359.6985, 83.1487) (-359.81, 83.1056) (-359.9166, 83.0639) (-359.9697, 83.043) knots -0.041525 -0.041525 -0.041525 -0.041525 -0.041525 -0.041525 -0.04 -0.02 0 0 0 0 0 0
  spline S7 degree 5 poles (-359.9697, 83.043) (-359.958, 82.9935) (-359.9278, 82.8821) (-359.8622, 82.6775) (-359.7337, 82.3297) (-359.5055, 81.771) (-359.2118, 81.0929) (-358.8574, 80.3045) (-358.4508, 79.4224) (-358.0035, 78.4687) (-357.5291, 77.4686) (-357.0428, 76.4482) (-356.5602, 75.4327) (-356.0968, 74.4439) (-355.6671, 73.4983) (-355.2837, 72.6045) (-354.9569, 71.7634) (-354.6951, 70.9706) (-354.5046, 70.219) (-354.3894, 69.5005) (-354.3516, 68.808) (-354.391, 68.1384) (-354.5054, 67.4925) (-354.6905, 66.8732) (-354.9403, 66.2847) (-355.2464, 65.7307) (-355.5989, 65.2134) (-355.9865, 64.7329) (-356.3978, 64.2876) (-356.8218, 63.8741) (-357.2495, 63.4874) (-357.674, 63.1207) (-358.0905, 62.7671) (-358.4957, 62.4196) (-358.8875, 62.0728) (-359.2647, 61.7233) (-359.5543, 61.4403) (-359.7646, 61.2258) (-359.9018, 61.0819) (-359.9697, 61.0097) knots -1 -1 -1 -1 -1 -1 -0.971429 -0.942857 -0.914286 -0.885714 -0.857143 -0.828571 -0.8 -0.771429 -0.742857 -0.714286 -0.685714 -0.657143 -0.628571 -0.6 -0.571429 -0.542857 -0.514286 -0.485714 -0.457143 -0.428571 -0.4 -0.371429 -0.342857 -0.314286 -0.285714 -0.257143 -0.228571 -0.2 -0.171429 -0.142857 -0.114286 -0.085714 -0.057143 -0.028571 0 0 0 0 0 0
  line L23 (-359.9697, 61.0097) -> (-359.9697, 35.6695)
  line L24 (-359.9697, 35.6695) -> (-332.3207, 27.7023)
  line L25 (-332.3207, 27.7023) -> (-325.7445, 21.4703)
  line L26 (-325.7445, 21.4703) -> (-326.0635, 21.1597)
  line L27 (-326.0635, 21.1597) -> (-333.1, 13.7167)
  spline S8 degree 5 poles (-333.1, 13.7167) (-333.3878, 13.6343) (-333.9657, 13.4696) (-334.8388, 13.2226) (-336.0158, 12.8932) (-337.5089, 12.4816) (-339.0245, 12.0695) (-340.5633, 11.6563) (-342.1264, 11.2407) (-343.7147, 10.8206) (-345.3286, 10.394) (-346.9663, 9.9592) (-348.6228, 9.5161) (-350.2888, 9.0666) (-351.9486, 8.6156) (-353.5804, 8.1713) (-355.1586, 7.7439) (-356.6573, 7.3442) (-358.0528, 6.9821) (-359.3264, 6.6655) (-360.4685, 6.3988) (-361.274, 6.2265) (-361.8173, 6.1205) (-362.1526, 6.0601) (-362.3136, 6.0325) knots -1 -1 -1 -1 -1 -1 -0.95 -0.9 -0.85 -0.8 -0.75 -0.7 -0.65 -0.6 -0.55 -0.5 -0.45 -0.4 -0.35 -0.3 -0.25 -0.2 -0.15 -0.1 -0.05 0 0 0 0 0 0
  line L28 (-407.924, 245) -> (-407.924, 0)
  line L29 (-407.924, 0) -> (-285.1, 0)
  line L30 (-285.1, 0) -> (-285.1, 220)
  line L31 (-285.1, 220) -> (-312.924, 220)
  line L32 (-312.924, 220) -> (-312.924, 245)
  line L33 (-312.924, 245) -> (-407.924, 245)
  line L34 (-289.1, 216) -> (-316.924, 216)
  line L35 (-316.924, 216) -> (-316.924, 241)
  line L36 (-316.924, 241) -> (-403.924, 241)
  line L37 (-403.924, 241) -> (-403.924, 4)
  line L38 (-403.924, 4) -> (-289.1, 4)
  line L39 (-289.1, 4) -> (-289.1, 216)
  line L40 (-289.1, 4) -> (-316.6, 4)
  line L41 (-316.6, 4) -> (-316.6, 214)
  line L42 (-316.6, 214) -> (-289.1, 214)
  line L43 (-289.1, 214) -> (-289.1, 4)
  dimension "d241" = 27.5
  dimension "d242" = 210
  constraint horizontal L40
  constraint vertical L41
  constraint horizontal L42
  constraint vertical L43
  measures "d241" distance of L38.end L40.end
  measures "d242" distance of L38.end L42.end
extrude "Extrude8" cut sketch "Sketch10" against normal blind 45 contours L38 L39 L40 L41 L42 L43
extrude "Extrude9" cut 1 faces at (294.3747, -220, 18.175) along direction (0, 1, 0) blind 2
extrude "Extrude10" [suppressed]
extrude "Extrude11" [suppressed]
extrude "Extrude12" [suppressed]
extrude "Extrude13" [suppressed]